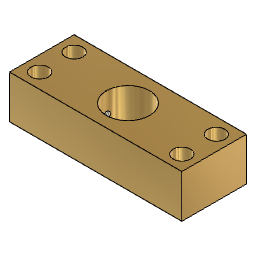
SeedMint assembly (Autodesk Fusion 360 archive; units mm, degrees)
design "Retainer"
Autodesk Fusion 360 part; units mm, degrees
sketch "Skizze1" plane through (0, 0, 0) normal (0, 0, 1) x (1, 0, 0)
  line L0 (0, 0) -> (80, 0)
  line L1 (80, 0) -> (80, 30)
  line L2 (80, 30) -> (0, 30)
  line L3 (0, 30) -> (0, 0)
  dimension "d1" = 80
  dimension "d2" = 30
  constraint horizontal L0
  constraint vertical L1
  constraint horizontal L2
  constraint vertical L3
  constraint coincident L0.start L3.end
  measures "d1" distance of L0.start L0.end
  measures "d2" distance of L0.start L2.end
extrude "Extrusion1" add sketch "Skizze1" along normal blind 20
sketch "Skizze2" plane through (0, 0, 20) normal (0, 0, 1) x (-1, 0, 0)
  line L0 (0, -30) -> (0, 0)
  line L1 (0, 0) -> (-80, 0)
  line L2 (-80, 0) -> (-80, -30)
  line L3 (-80, -30) -> (0, -30)
  circle A0 centre (-40, -15) radius 10
  circle A1 centre (-7, -23) radius 2.5
  circle A2 centre (-7, -23) radius 4
  dimension "d5" = 20
  dimension "d6" = 40
  dimension "d7" = 15
  dimension "d8" = 5
  dimension "d9" = 8
  dimension "d10" = 7
  dimension "d11" = 7
  constraint concentric A1 A2
  measures "d5" diameter of A0
  measures "d6" distance of L0 A0.centre
  measures "d7" distance of L1 A0.centre
  measures "d8" diameter of A1
  measures "d9" diameter of A2
  measures "d10" distance of L0 A1.centre
  measures "d11" distance of L3 A1.centre
extrude "Extrusion2" cut sketch "Skizze2" against normal blind 22 contours A0
ref_plane "Arbeitsebene1" through (40, 15, 10) normal (0, -1, 0) x (1, 0, 0)
extrude "Extrusion3" cut sketch "Skizze2" against normal blind 22 contours A1
extrude "Extrusion4" cut sketch "Skizze2" against normal blind 7 contours A2
pattern_linear "R-Anordnung1" count 2 spacing 16 along (0, -1, 0) count 2 spacing 66 along (1, 0, 0) of "Extrusion3", "Extrusion4"
sketch "Skizze3" plane through (0, 0, 0) normal (-1, 0, 0) x (0, -1, 0)
  line L0 (-30, 0) -> (0, 0)
  line L1 (0, 0) -> (0, 20)
  line L2 (0, 20) -> (-30, 20)
  line L3 (-30, 20) -> (-30, 0)
  circle A0 centre (-15, 10) radius 1.5
  dimension "d22" = 3
  dimension "d23" = 15
  dimension "d24" = 10
  measures "d22" diameter of A0
  measures "d23" distance of L3 A0.centre
  measures "d24" distance of L0 A0.centre
hole "Bohrung1" at (0, 15, 10) direction (1, 0, 0) diameter 3.332 depth 40 tip angle 118
thread "Gewinde3" "ISO Metric profile 4.0 M4x0.7 6H"
chamfer "Fase3" distance 0.3 angle 45 1 edges at (0, 16.5533, 10.6025)

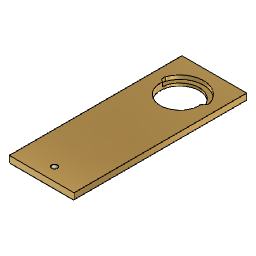
design "Slider"
Autodesk Fusion 360 part; units mm, degrees
sketch "Skizze1" plane through (0, 0, 0) normal (0, 0, 1) x (1, 0, 0)
  line L0 (0, 0) -> (30, 0)
  line L1 (30, 0) -> (30, 80)
  line L2 (30, 80) -> (0, 80)
  line L3 (0, 80) -> (0, 0)
  dimension "d1" = 80
  dimension "d2" = 30
  constraint horizontal L0
  constraint vertical L1
  constraint horizontal L2
  constraint vertical L3
  constraint coincident L0.start L3.end
  measures "d1" distance of L0.start L2.end
  measures "d2" distance of L1 L3
extrude "Extrusion1" add sketch "Skizze1" along normal blind 3
sketch "Skizze2" plane through (0, 0, 3) normal (0, 0, 1) x (-1, 0, 0)
  line L0 (0, -80) -> (0, 0)
  line L1 (0, 0) -> (-30, 0)
  line L2 (-30, 0) -> (-30, -80)
  line L3 (-30, -80) -> (0, -80)
  circle A0 centre (-15, -64) radius 9
  circle A1 centre (-15, -64) radius 11
  circle A2 centre (-15, -6) radius 1.5
  arc A3 (-4.1818, -62.0083) -> (-4.1818, -65.9917) centre (-4, -64) ccw
  arc A4 (-25.8182, -65.9917) -> (-25.8182, -62.0083) centre (-26, -64) ccw
  line L4 (-4.1818, -65.9917) -> (-15, -60)
  line L5 (-15, -60) -> (-25.8182, -65.9917)
  point P0 (-15, -60)
  dimension "d5" = 18
  dimension "d6" = 64
  dimension "d7" = 22
  dimension "d8" = 64
  dimension "d9" = 15
  dimension "d10" = 3
  dimension "d11" = 6
  dimension "d26" = 4
  dimension "d27" = 4
  dimension "d36" = 4
  constraint vertical A0.centre A1.centre
  constraint vertical A0.centre A2.centre
  constraint coincident A1 A4.centre
  constraint coincident A1 A3.centre
  constraint horizontal A0.centre A3.centre
  constraint horizontal A0.centre A4.centre
  constraint coincident A1 A3.end
  constraint coincident A1 A3.start
  constraint coincident A1 A4.end
  constraint coincident A1 A4.start
  constraint vertical A0.centre P0
  constraint coincident P0 L4.end
  measures "d5" diameter of A0
  measures "d6" distance of L1 A0.centre
  measures "d7" diameter of A1
  measures "d8" distance of L1 A0.centre
  measures "d9" distance of L0 A0.centre
  measures "d10" diameter of A2
  measures "d11" distance of L1 A2.centre
  measures "d26" diameter of A4
  measures "d27" diameter of A3
  measures "d36" distance of A0.centre P0
extrude "Extrusion2" cut sketch "Skizze2" against normal blind 4 contours A0 L4 L5 | A0 L4 L5
extrude "Extrusion3" cut sketch "Skizze2" against normal blind 1.8 contours A0 A3 L4 | A0 A1 A3 A4 | A1 A3 L4 | A0 A4 L5 | A1 A4 L5 | A0 A1 A3 A4 L4 L5 | A3 L4 | A4 L5
extrude "Extrusion4" cut sketch "Skizze2" against normal blind 4 contours A2
thread "Gewinde1" "ISO Metric profile 3.0 M3x0.5 6H" major diameter 3.086 minor diameter 2.529 pitch 0.5 angle 60 resizes the face on face at (13.5075, 6.1494, 2)
chamfer "Fase1" distance 0.1 angle 45 1 edges at (16.1789, 5.5427, 3)
sketch "Skizze3" plane through (0, 0, 0) normal (0, 0, -1) x (1, 0, 0)
  circle A0 centre (15, -6) radius 1.2645
  circle A1 centre (15, -64) radius 9
  line L0 (0, 0) -> (0, -80)
  line L1 (0, -80) -> (30, -80)
  line L2 (30, -80) -> (30, 0)
  line L3 (30, 0) -> (0, 0)
  line L4 (17, -46) -> (17, -17)
  arc A2 (17, -17) -> (13, -17) centre (15, -17) ccw
  line L5 (13, -17) -> (13, -46)
  arc A3 (13, -46) -> (17, -46) centre (15, -46) ccw
  line L6 (15, -48) -> (15, -15) construction
  dimension "d19" = 4
  dimension "d20" = 15
  dimension "d21" = 33
  dimension "d22" = 15
  constraint tangent L4 A2
  constraint tangent A2 L5
  constraint parallel L4 L5
  constraint tangent L5 A3
  constraint tangent L4 A3
  constraint midpoint A3 L6.start
  constraint midpoint A2 L6.end
  constraint parallel L2 L6
  measures "d19" diameter of A2
  measures "d20" distance of L3 L6.end
  measures "d21" distance of L6.start L6.end
  measures "d22" distance of L2 L6
extrude "Extrusion5" cut sketch "Skizze3" against normal blind 2 contours L4 A2 L5 A3
chamfer "Fase2" distance 0.2 angle 45 2 edges at (0, 40, 0) (30, 40, 0)
extrude "Extrusion9" add sketch "Skizze2" against normal blind 1.8 contours A0 A3 L4 | A0 A1 A3 A4 | A1 A3 L4 | A0 A4 L5 | A1 A4 L5
fillet "Abrundung2" radius 2 2 edges at (25.8182, 65.9917, 2.1) (4.1818, 65.9917, 2.1)
sketch "Skizze4" plane through (0, 0, 3) normal (0, 0, 1) x (-1, 0, 0)
  arc A0 (-25.376, -67.6522) -> (-4.624, -67.6522) centre (-15, -64) ccw
  line L0 (-5.5415, -65.2386) -> (-6.051, -64.9565)
  line L1 (-23.949, -64.9565) -> (-24.4585, -65.2386)
  circle A1 centre (-15, -64) radius 11
  line L2 (-15, -60) -> (-25.8182, -65.9917)
  line L3 (-4.1818, -65.9917) -> (-15, -60)
  constraint concentric A0 A1
  constraint coincident A0.start A1
  constraint coincident A1 L2.end
  constraint collinear L1 L2
  constraint coincident A1 L3.start
  constraint collinear L0 L3
sketch "Skizze5" plane through (0, 0, 3) normal (0, 0, 1) x (-1, 0, 0)
  line L0 (0, -80) -> (0, 0)
  line L1 (0, 0) -> (-30, 0)
  line L2 (-30, 0) -> (-30, -80)
  line L3 (-30, -80) -> (0, -80)
  arc A0 (-25.376, -67.6522) -> (-4.624, -67.6522) centre (-15, -64) ccw
  arc A1 (-24.4585, -65.2386) -> (-25.376, -67.6522) centre (-23.4894, -66.9882) ccw
  line L4 (-24.4585, -65.2386) -> (-23.949, -64.9565)
  arc A2 (-6.051, -64.9565) -> (-23.949, -64.9565) centre (-15, -64) ccw
  line L5 (-6.051, -64.9565) -> (-5.5415, -65.2386)
  arc A3 (-4.624, -67.6522) -> (-5.5415, -65.2386) centre (-6.5106, -66.9882) ccw
  circle A4 centre (-15, -6) radius 1.3645
  point P0 (-4.1818, -65.9917)
  point P1 (-25.8182, -65.9917)
  point P2 (-15, -60)
equation "d8 = d6"
